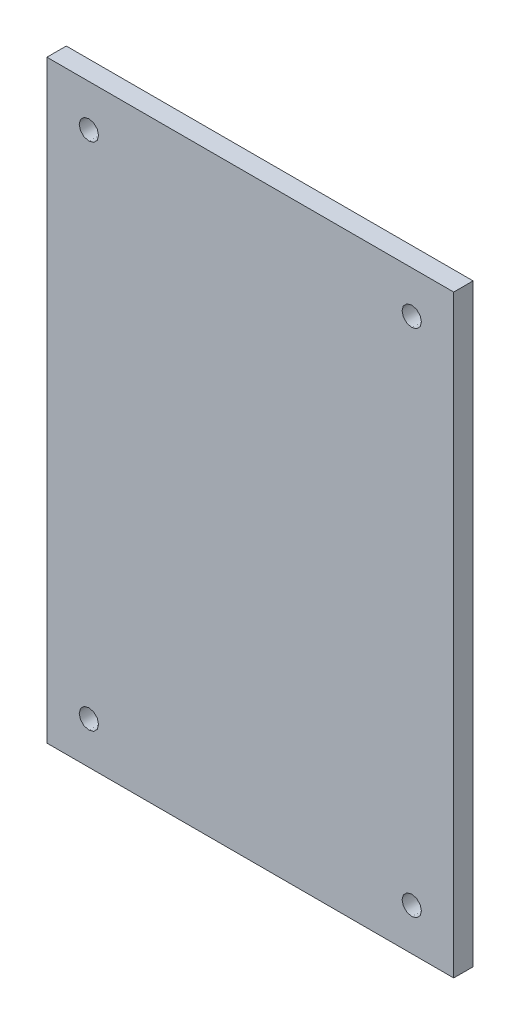
# Autodesk Inventor part: base teclado
Saved by Autodesk Inventor 2017 (Build 210142000, 142)
## iProperties
Created: 2017-08-05
Part Number: base teclado
Material: Generic
Document SubType Name: Modeling
Designer: leo
Density: 1 g/cm^3
Appearance: Default
Author: leo
Autodesk Inventor part; units mm, degrees
ref_plane "YZ Plane" through (0, 0, 0) normal (1, 0, 0) x (0, 1, 0)
ref_plane "XZ Plane" through (0, 0, 0) normal (0, 1, 0) x (-1, 0, 0)
ref_plane "XY Plane" through (0, 0, 0) normal (0, 0, 1) x (1, 0, 0)
sketch "Sketch1" plane through (0, 0, 0) normal (0, 0, 1) x (1, 0, 0)
  line L0 (31.5, 48.5) -> (31.5, -43.5)
  line L1 (31.5, -43.5) -> (-31.5, -43.5)
  line L2 (-31.5, -43.5) -> (-31.5, 48.5)
  line L3 (-31.5, 48.5) -> (31.5, 48.5)
  line L4 (25, -37) -> (25, 42) construction
  line L5 (25, 42) -> (-25, 42) construction
  line L6 (-25, 42) -> (-25, -37) construction
  line L7 (-25, -37) -> (25, -37) construction
  circle A0 centre (25, 42) radius 1.5 projected
  circle A1 centre (25, -37) radius 1.5 projected
  circle A2 centre (-25, -37) radius 1.5 projected
  circle A3 centre (-25, 42) radius 1.5 projected
  point P0 (0, 0)
  dimension "d0" = 5
  constraints: 16 end point, 6 perpendicular, 2 coincident, 1 vertical, 3 other
  measures "d0" distance edge to line of A0 L0
extrude "Extrusion1" add sketch "Sketch1" along normal blind 3
body "Solid1"
